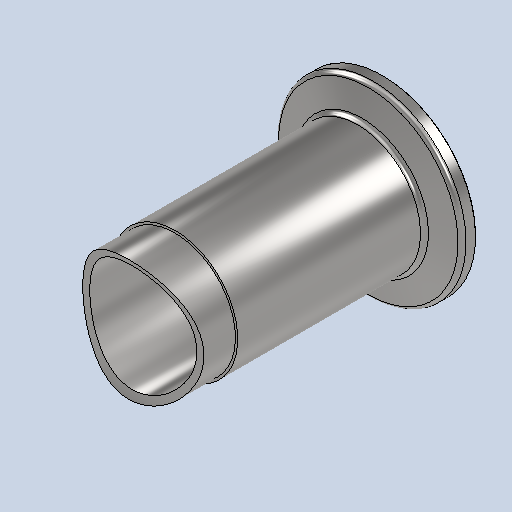
# Autodesk Inventor part: pld_vessel_kf_nipple
Saved by Autodesk Inventor 2026 (Build 300175050, 175E)
## iProperties
Created: 2025-11-13
Part Number: pld_vessel_kf_nipple
Material: Stainless Steel
Document SubType Name: Modeling
Designer: kuzmin
Density: 8 g/cm^3
Appearance: Semi-Polished
Author: kuzmin
Autodesk Inventor part; units mm, degrees
ref_plane "YZ Plane" through (0, 0, 0) normal (1, 0, 0) x (0, 1, 0)
ref_plane "XZ Plane" through (0, 0, 0) normal (0, 1, 0) x (-1, 0, 0)
ref_plane "XY Plane" through (0, 0, 0) normal (0, 0, 1) x (1, 0, 0)
sketch "Sketch1" plane through (0, 0, 0) normal (1, 0, 0) x (0, 1, 0)
  line L0 (0, 0) -> (0, 56)
  line L1 (-11.5, 56) -> (-11.5, 2.5)
  line L2 (-11.5, 2.5) -> (-13, 2.5)
  line L3 (-13, 2.5) -> (-13, 0)
  line L4 (-13, 0) -> (-20, 0)
  line L5 (-20, 0) -> (-20, 3)
  line L6 (-20, 3) -> (-13.5, 4.7417)
  line L7 (-13.5, 4.7417) -> (-13.5, 44.7417)
  line L8 (-13.5, 44.7417) -> (-13, 44.7417)
  line L9 (-13, 44.7417) -> (-13, 56)
  line L10 (-13, 56) -> (-11.5, 56)
  dimension "d0" = 56
  dimension "d1" = 27
  dimension "d2" = 26
  dimension "d3" = 2.5
  dimension "d4" = 23
  dimension "d5" = 15
  dimension "d6" = 3
  dimension "d7" = 40
  dimension "d8" = 26
  dimension "d10" = 40
  constraints: 22 end point, 7 perpendicular, 2 horizontal alignment, 2 vertical, 1 parallel
  measures "d0" distance of L0.start L0.end
  measures "d1" diameter of L7 L0
  measures "d2" diameter of L3 L0
  measures "d3" distance of L2.end L3.end
  measures "d4" diameter of L1 L0
  measures "d5" angle of L2 L6
  measures "d6" distance of L4.end L5.end
  measures "d7" diameter of L5 L0
  measures "d8" diameter of L9 L0
  measures "d10" distance of L6.end L7.end
revolve "Revolution1" add sketch "Sketch1" angle 360 about axis through (0, 0, 0) along (0, 0, 1)
fillet "Fillet1" radius 1 2 edges at (0, 20, 3) (0, 13.5, 4.7417)
sketch "Sketch2" plane through (0, 0, 0) normal (1, 0, 0) x (0, 1, 0)
  circle A0 centre (0, 80) radius 28.5
  line L0 (20, 0) -> (-20, 0) projected
  point P0 (0, 0)
  dimension "d13" = 57
  dimension "d14" = 80
  constraints: 1 centre point
  measures "d13" diameter of A0
  measures "d14" distance from line of L0 A0.centre
extrude "Extrusion1" cut sketch "Sketch2" along normal through all both and the other way through all
chamfer "Chamfer1" distance 0.2 angle 45 4 edges at (0, 20, 0) (0, 13, 0) (0, 11.5, 2.5) (0, 13, 2.5)
body "Solid1"
